Autodesk Fusion 360 part; units mm, degrees
(part 4 of 6)
sketch "Sketch2" plane through (0, 0, 0) normal (0, 0, -1) x (1, 0, 0)
  line L0 (-67.0711, -60) -> (-70, -62.9289)
  line L1 (-70, -62.9289) -> (-70, -57.0711)
  line L2 (-70, -57.0711) -> (-67.0711, -60)
  line L3 (-62.9289, -60) -> (-60, -57.0711)
  line L4 (-60, -57.0711) -> (-57.0711, -60)
  line L5 (-57.0711, -60) -> (-60, -62.9289)
  line L6 (-60, -62.9289) -> (-62.9289, -60)
  line L7 (-60, -67.0711) -> (-57.0711, -70)
  line L8 (-57.0711, -70) -> (-62.9289, -70)
  line L9 (-62.9289, -70) -> (-60, -67.0711)
  line L10 (-52.9289, -70) -> (-50, -67.0711)
  line L11 (-50, -67.0711) -> (-47.0711, -70)
  line L12 (-47.0711, -70) -> (-52.9289, -70)
  line L13 (-42.9289, -70) -> (-40, -67.0711)
  line L14 (-40, -67.0711) -> (-37.0711, -70)
  line L15 (-37.0711, -70) -> (-42.9289, -70)
  line L16 (-32.9289, -70) -> (-30, -67.0711)
  line L17 (-30, -67.0711) -> (-27.0711, -70)
  line L18 (-27.0711, -70) -> (-32.9289, -70)
  line L19 (-22.9289, -70) -> (-20, -67.0711)
  line L20 (-20, -67.0711) -> (-17.0711, -70)
  line L21 (-17.0711, -70) -> (-22.9289, -70)
  line L22 (-12.9289, -70) -> (-10, -67.0711)
  line L23 (-10, -67.0711) -> (-7.0711, -70)
  line L24 (-7.0711, -70) -> (-12.9289, -70)
  line L25 (-2.9289, -70) -> (0, -67.0711)
  line L26 (0, -67.0711) -> (2.9289, -70)
  line L27 (2.9289, -70) -> (-2.9289, -70)
  line L28 (7.0711, -70) -> (10, -67.0711)
  line L29 (10, -67.0711) -> (12.9289, -70)
  line L30 (12.9289, -70) -> (7.0711, -70)
  line L31 (17.0711, -70) -> (20, -67.0711)
  line L32 (20, -67.0711) -> (22.9289, -70)
  line L33 (22.9289, -70) -> (17.0711, -70)
  line L34 (27.0711, -70) -> (30, -67.0711)
  line L35 (30, -67.0711) -> (32.9289, -70)
  line L36 (32.9289, -70) -> (27.0711, -70)
  line L37 (37.0711, -70) -> (40, -67.0711)
  line L38 (40, -67.0711) -> (42.9289, -70)
  line L39 (42.9289, -70) -> (37.0711, -70)
  line L40 (47.0711, -70) -> (50, -67.0711)
  line L41 (50, -67.0711) -> (52.9289, -70)
  line L42 (52.9289, -70) -> (47.0711, -70)
  line L43 (57.0711, -70) -> (60, -67.0711)
  line L44 (60, -67.0711) -> (62.9289, -70)
  line L45 (62.9289, -70) -> (57.0711, -70)
  line L46 (67.0711, -70) -> (70, -67.0711)
  line L47 (70, -67.0711) -> (70, -70)
  line L48 (70, -70) -> (67.0711, -70)
  line L49 (70, -62.9289) -> (67.0711, -60)
  line L50 (67.0711, -60) -> (70, -57.0711)
  line L51 (70, -57.0711) -> (70, -62.9289)
  line L52 (70, -52.9289) -> (67.0711, -50)
  line L53 (67.0711, -50) -> (70, -47.0711)
  line L54 (70, -47.0711) -> (70, -52.9289)
  line L55 (70, -42.9289) -> (67.0711, -40)
  line L56 (67.0711, -40) -> (70, -37.0711)
  line L57 (70, -37.0711) -> (70, -42.9289)
  line L58 (70, -32.9289) -> (67.0711, -30)
  line L59 (67.0711, -30) -> (70, -27.0711)
  line L60 (70, -27.0711) -> (70, -32.9289)
  line L61 (70, -22.9289) -> (67.0711, -20)
  line L62 (67.0711, -20) -> (70, -17.0711)
  line L63 (70, -17.0711) -> (70, -22.9289)
  line L64 (70, -12.9289) -> (67.0711, -10)
  line L65 (67.0711, -10) -> (70, -7.0711)
  line L66 (70, -7.0711) -> (70, -12.9289)
  line L67 (70, -2.9289) -> (67.0711, 0)
  line L68 (67.0711, 0) -> (70, 2.9289)
  line L69 (70, 2.9289) -> (70, -2.9289)
  line L70 (70, 7.0711) -> (67.0711, 10)
  line L71 (67.0711, 10) -> (70, 12.9289)
  line L72 (70, 12.9289) -> (70, 7.0711)
  line L73 (70, 17.0711) -> (67.0711, 20)
  line L74 (67.0711, 20) -> (70, 22.9289)
  line L75 (70, 22.9289) -> (70, 17.0711)
  line L76 (70, 27.0711) -> (67.0711, 30)
  line L77 (67.0711, 30) -> (70, 32.9289)
  line L78 (70, 32.9289) -> (70, 27.0711)
  line L79 (70, 37.0711) -> (67.0711, 40)
  line L80 (67.0711, 40) -> (70, 42.9289)
  line L81 (70, 42.9289) -> (70, 37.0711)
  line L82 (70, 47.0711) -> (67.0711, 50)
  line L83 (67.0711, 50) -> (70, 52.9289)
  line L84 (70, 52.9289) -> (70, 47.0711)
  line L85 (70, 57.0711) -> (67.0711, 60)
  line L86 (67.0711, 60) -> (70, 62.9289)
  line L87 (70, 62.9289) -> (70, 57.0711)
  line L88 (70, 67.0711) -> (67.0711, 70)
  line L89 (67.0711, 70) -> (70, 70)
  line L90 (70, 70) -> (70, 67.0711)
  line L91 (62.9289, 70) -> (60, 67.0711)
  line L92 (60, 67.0711) -> (57.0711, 70)
  line L93 (57.0711, 70) -> (62.9289, 70)
  line L94 (52.9289, 70) -> (50, 67.0711)
  line L95 (50, 67.0711) -> (47.0711, 70)
  line L96 (47.0711, 70) -> (52.9289, 70)
  line L97 (42.9289, 70) -> (40, 67.0711)
  line L98 (40, 67.0711) -> (37.0711, 70)
  line L99 (37.0711, 70) -> (42.9289, 70)
  line L100 (32.9289, 70) -> (30, 67.0711)
  line L101 (30, 67.0711) -> (27.0711, 70)
  line L102 (27.0711, 70) -> (32.9289, 70)
  line L103 (22.9289, 70) -> (20, 67.0711)
  line L104 (20, 67.0711) -> (17.0711, 70)
  line L105 (17.0711, 70) -> (22.9289, 70)
  line L106 (12.9289, 70) -> (10, 67.0711)
  line L107 (10, 67.0711) -> (7.0711, 70)
  line L108 (7.0711, 70) -> (12.9289, 70)
  line L109 (2.9289, 70) -> (0, 67.0711)
  line L110 (0, 67.0711) -> (-2.9289, 70)
  line L111 (-2.9289, 70) -> (2.9289, 70)
  line L112 (-7.0711, 70) -> (-10, 67.0711)
  line L113 (-10, 67.0711) -> (-12.9289, 70)
  line L114 (-12.9289, 70) -> (-7.0711, 70)
  line L115 (-17.0711, 70) -> (-20, 67.0711)
  line L116 (-20, 67.0711) -> (-22.9289, 70)
  line L117 (-22.9289, 70) -> (-17.0711, 70)
  line L118 (-27.0711, 70) -> (-30, 67.0711)
  line L119 (-30, 67.0711) -> (-32.9289, 70)
  line L120 (-32.9289, 70) -> (-27.0711, 70)
  line L121 (-37.0711, 70) -> (-40, 67.0711)
  line L122 (-40, 67.0711) -> (-42.9289, 70)
  line L123 (-42.9289, 70) -> (-37.0711, 70)
  line L124 (-47.0711, 70) -> (-50, 67.0711)
  line L125 (-50, 67.0711) -> (-52.9289, 70)
  line L126 (-52.9289, 70) -> (-47.0711, 70)
  line L127 (-57.0711, 70) -> (-60, 67.0711)
  line L128 (-60, 67.0711) -> (-62.9289, 70)
  line L129 (-62.9289, 70) -> (-57.0711, 70)
  line L130 (-67.0711, 70) -> (-70, 67.0711)
  line L131 (-70, 67.0711) -> (-70, 70)
  line L132 (-70, 70) -> (-67.0711, 70)
  line L133 (-70, 62.9289) -> (-67.0711, 60)
  line L134 (-67.0711, 60) -> (-70, 57.0711)
  line L135 (-70, 57.0711) -> (-70, 62.9289)
  line L136 (-70, 52.9289) -> (-67.0711, 50)
  line L137 (-67.0711, 50) -> (-70, 47.0711)
  line L138 (-70, 47.0711) -> (-70, 52.9289)
  line L139 (-70, 42.9289) -> (-67.0711, 40)
  line L140 (-67.0711, 40) -> (-70, 37.0711)
  line L141 (-70, 37.0711) -> (-70, 42.9289)
  line L142 (-70, 32.9289) -> (-67.0711, 30)
  line L143 (-67.0711, 30) -> (-70, 27.0711)
  line L144 (-70, 27.0711) -> (-70, 32.9289)
  line L145 (-70, 22.9289) -> (-67.0711, 20)
  line L146 (-67.0711, 20) -> (-70, 17.0711)
  line L147 (-70, 17.0711) -> (-70, 22.9289)
  line L148 (-70, 12.9289) -> (-67.0711, 10)
  line L149 (-67.0711, 10) -> (-70, 7.0711)
  line L150 (-70, 7.0711) -> (-70, 12.9289)
  line L151 (-70, 2.9289) -> (-67.0711, 0)
  line L152 (-67.0711, 0) -> (-70, -2.9289)
  line L153 (-70, -2.9289) -> (-70, 2.9289)
  line L154 (-70, -7.0711) -> (-67.0711, -10)
  line L155 (-67.0711, -10) -> (-70, -12.9289)
  line L156 (-70, -12.9289) -> (-70, -7.0711)
  line L157 (-70, -17.0711) -> (-67.0711, -20)
  line L158 (-67.0711, -20) -> (-70, -22.9289)
  line L159 (-70, -22.9289) -> (-70, -17.0711)
  line L160 (-70, -27.0711) -> (-67.0711, -30)
  line L161 (-67.0711, -30) -> (-70, -32.9289)
  line L162 (-70, -32.9289) -> (-70, -27.0711)
  line L163 (-70, -37.0711) -> (-67.0711, -40)
  line L164 (-67.0711, -40) -> (-70, -42.9289)
  line L165 (-70, -42.9289) -> (-70, -37.0711)
  line L166 (-17.0711, 40) -> (-20, 37.0711)
  line L167 (-20, 37.0711) -> (-22.9289, 40)
  line L168 (-22.9289, 40) -> (-20, 42.9289)
  line L169 (-20, 42.9289) -> (-17.0711, 40)
  line L170 (-27.0711, 40) -> (-30, 37.0711)
  line L171 (-30, 37.0711) -> (-32.9289, 40)
  line L172 (-32.9289, 40) -> (-30, 42.9289)
  line L173 (-30, 42.9289) -> (-27.0711, 40)
  line L174 (-37.0711, 40) -> (-40, 37.0711)
  line L175 (-40, 37.0711) -> (-42.9289, 40)
  line L176 (-42.9289, 40) -> (-40, 42.9289)
  line L177 (-40, 42.9289) -> (-37.0711, 40)
  line L178 (-37.0711, 30) -> (-40, 27.0711)
  line L179 (-40, 27.0711) -> (-42.9289, 30)
  line L180 (-42.9289, 30) -> (-40, 32.9289)
  line L181 (-40, 32.9289) -> (-37.0711, 30)
  line L182 (-37.0711, 20) -> (-40, 17.0711)
  line L183 (-40, 17.0711) -> (-42.9289, 20)
  line L184 (-42.9289, 20) -> (-40, 22.9289)
  line L185 (-40, 22.9289) -> (-37.0711, 20)
  line L186 (-37.0711, 10) -> (-40, 7.0711)
  line L187 (-40, 7.0711) -> (-42.9289, 10)
  line L188 (-42.9289, 10) -> (-40, 12.9289)
  line L189 (-40, 12.9289) -> (-37.0711, 10)
  line L190 (-37.0711, 0) -> (-40, -2.9289)
  line L191 (-40, -2.9289) -> (-42.9289, 0)
  line L192 (-42.9289, 0) -> (-40, 2.9289)
  line L193 (-40, 2.9289) -> (-37.0711, 0)
  line L194 (-37.0711, -10) -> (-40, -12.9289)
  line L195 (-40, -12.9289) -> (-42.9289, -10)
  line L196 (-42.9289, -10) -> (-40, -7.0711)
  line L197 (-40, -7.0711) -> (-37.0711, -10)
  line L198 (-37.0711, -20) -> (-40, -22.9289)
  line L199 (-40, -22.9289) -> (-42.9289, -20)
  line L200 (-42.9289, -20) -> (-40, -17.0711)
  line L201 (-40, -17.0711) -> (-37.0711, -20)
  line L202 (-37.0711, -30) -> (-40, -32.9289)
  line L203 (-40, -32.9289) -> (-42.9289, -30)
  line L204 (-42.9289, -30) -> (-40, -27.0711)
  line L205 (-40, -27.0711) -> (-37.0711, -30)
  line L206 (-27.0711, -20) -> (-30, -22.9289)
  line L207 (-30, -22.9289) -> (-32.9289, -20)
  line L208 (-32.9289, -20) -> (-30, -17.0711)
  line L209 (-30, -17.0711) -> (-27.0711, -20)
  line L210 (-17.0711, -20) -> (-20, -22.9289)
  line L211 (-20, -22.9289) -> (-22.9289, -20)
  line L212 (-22.9289, -20) -> (-20, -17.0711)
  line L213 (-20, -17.0711) -> (-17.0711, -20)
  line L214 (-7.0711, -30) -> (-10, -32.9289)
  line L215 (-10, -32.9289) -> (-12.9289, -30)
  line L216 (-12.9289, -30) -> (-10, -27.0711)
  line L217 (-10, -27.0711) -> (-7.0711, -30)
  line L218 (2.9289, -30) -> (0, -32.9289)
  line L219 (0, -32.9289) -> (-2.9289, -30)
  line L220 (-2.9289, -30) -> (0, -27.0711)
  line L221 (0, -27.0711) -> (2.9289, -30)
  line L222 (12.9289, -30) -> (10, -32.9289)
  line L223 (10, -32.9289) -> (7.0711, -30)
  line L224 (7.0711, -30) -> (10, -27.0711)
  line L225 (10, -27.0711) -> (12.9289, -30)
  line L226 (22.9289, -30) -> (20, -32.9289)
  line L227 (20, -32.9289) -> (17.0711, -30)
  line L228 (17.0711, -30) -> (20, -27.0711)
  line L229 (20, -27.0711) -> (22.9289, -30)
  line L230 (32.9289, -30) -> (30, -32.9289)
  line L231 (30, -32.9289) -> (27.0711, -30)
  line L232 (27.0711, -30) -> (30, -27.0711)
  line L233 (30, -27.0711) -> (32.9289, -30)
  line L234 (32.9289, -10) -> (30, -12.9289)
  line L235 (30, -12.9289) -> (27.0711, -10)
  line L236 (27.0711, -10) -> (30, -7.0711)
  line L237 (30, -7.0711) -> (32.9289, -10)
  line L238 (32.9289, -20) -> (30, -22.9289)
  line L239 (30, -22.9289) -> (27.0711, -20)
  line L240 (27.0711, -20) -> (30, -17.0711)
  line L241 (30, -17.0711) -> (32.9289, -20)
  line L242 (32.9289, 10) -> (30, 7.0711)
  line L243 (30, 7.0711) -> (27.0711, 10)
  line L244 (27.0711, 10) -> (30, 12.9289)
  line L245 (30, 12.9289) -> (32.9289, 10)
  line L246 (32.9289, 20) -> (30, 17.0711)
  line L247 (30, 17.0711) -> (27.0711, 20)
  line L248 (27.0711, 20) -> (30, 22.9289)
  line L249 (30, 22.9289) -> (32.9289, 20)
  line L250 (32.9289, 0) -> (30, -2.9289)
  line L251 (30, -2.9289) -> (27.0711, 0)
  line L252 (27.0711, 0) -> (30, 2.9289)
  line L253 (30, 2.9289) -> (32.9289, 0)
  line L254 (32.9289, 30) -> (30, 27.0711)
  line L255 (30, 27.0711) -> (27.0711, 30)
  line L256 (27.0711, 30) -> (30, 32.9289)
  line L257 (30, 32.9289) -> (32.9289, 30)
  line L258 (12.9289, 30) -> (10, 27.0711)
  line L259 (10, 27.0711) -> (7.0711, 30)
  line L260 (7.0711, 30) -> (10, 32.9289)
  line L261 (10, 32.9289) -> (12.9289, 30)
  line L262 (2.9289, 30) -> (0, 27.0711)
  line L263 (0, 27.0711) -> (-2.9289, 30)
  line L264 (-2.9289, 30) -> (0, 32.9289)
  line L265 (0, 32.9289) -> (2.9289, 30)
  line L266 (-17.0711, 30) -> (-20, 27.0711)
  line L267 (-20, 27.0711) -> (-22.9289, 30)
  line L268 (-22.9289, 30) -> (-20, 32.9289)
  line L269 (-20, 32.9289) -> (-17.0711, 30)
  line L270 (-7.0711, 30) -> (-10, 27.0711)
  line L271 (-10, 27.0711) -> (-12.9289, 30)
  line L272 (-12.9289, 30) -> (-10, 32.9289)
  line L273 (-10, 32.9289) -> (-7.0711, 30)
  line L274 (-27.0711, 20) -> (-30, 17.0711)
  line L275 (-30, 17.0711) -> (-32.9289, 20)
  line L276 (-32.9289, 20) -> (-30, 22.9289)
  line L277 (-30, 22.9289) -> (-27.0711, 20)
  line L278 (-27.0711, 10) -> (-30, 7.0711)
  line L279 (-30, 7.0711) -> (-32.9289, 10)
  line L280 (-32.9289, 10) -> (-30, 12.9289)
  line L281 (-30, 12.9289) -> (-27.0711, 10)
  line L282 (-27.0711, 30) -> (-30, 27.0711)
  line L283 (-30, 27.0711) -> (-32.9289, 30)
  line L284 (-32.9289, 30) -> (-30, 32.9289)
  line L285 (-30, 32.9289) -> (-27.0711, 30)
  line L286 (-27.0711, 0) -> (-30, -2.9289)
  line L287 (-30, -2.9289) -> (-32.9289, 0)
  line L288 (-32.9289, 0) -> (-30, 2.9289)
  line L289 (-30, 2.9289) -> (-27.0711, 0)
  line L290 (-27.0711, -10) -> (-30, -12.9289)
  line L291 (-30, -12.9289) -> (-32.9289, -10)
  line L292 (-32.9289, -10) -> (-30, -7.0711)
  line L293 (-30, -7.0711) -> (-27.0711, -10)
  line L294 (-17.0711, -10) -> (-20, -12.9289)
  line L295 (-20, -12.9289) -> (-22.9289, -10)
  line L296 (-22.9289, -10) -> (-20, -7.0711)
  line L297 (-20, -7.0711) -> (-17.0711, -10)
  line L298 (-7.0711, -20) -> (-10, -22.9289)
  line L299 (-10, -22.9289) -> (-12.9289, -20)
  line L300 (-12.9289, -20) -> (-10, -17.0711)
  line L301 (-10, -17.0711) -> (-7.0711, -20)
  line L302 (2.9289, -20) -> (0, -22.9289)
  line L303 (0, -22.9289) -> (-2.9289, -20)
  line L304 (-2.9289, -20) -> (0, -17.0711)
  line L305 (0, -17.0711) -> (2.9289, -20)
  line L306 (12.9289, -20) -> (10, -22.9289)
  line L307 (10, -22.9289) -> (7.0711, -20)
  line L308 (7.0711, -20) -> (10, -17.0711)
  line L309 (10, -17.0711) -> (12.9289, -20)
  line L310 (22.9289, -20) -> (20, -22.9289)
  line L311 (20, -22.9289) -> (17.0711, -20)
  line L312 (17.0711, -20) -> (20, -17.0711)
  line L313 (20, -17.0711) -> (22.9289, -20)
  line L314 (22.9289, -10) -> (20, -12.9289)
  line L315 (20, -12.9289) -> (17.0711, -10)
  line L316 (17.0711, -10) -> (20, -7.0711)
  line L317 (20, -7.0711) -> (22.9289, -10)
  line L318 (22.9289, 10) -> (20, 7.0711)
  line L319 (20, 7.0711) -> (17.0711, 10)
  line L320 (17.0711, 10) -> (20, 12.9289)
  line L321 (20, 12.9289) -> (22.9289, 10)
  line L322 (22.9289, 20) -> (20, 17.0711)
  line L323 (20, 17.0711) -> (17.0711, 20)
  line L324 (17.0711, 20) -> (20, 22.9289)
  line L325 (20, 22.9289) -> (22.9289, 20)
  line L326 (22.9289, 0) -> (20, -2.9289)
  line L327 (20, -2.9289) -> (17.0711, 0)
  line L328 (17.0711, 0) -> (20, 2.9289)
  line L329 (20, 2.9289) -> (22.9289, 0)
  line L330 (22.9289, 30) -> (20, 27.0711)
  line L331 (20, 27.0711) -> (17.0711, 30)
  line L332 (17.0711, 30) -> (20, 32.9289)
  line L333 (20, 32.9289) -> (22.9289, 30)
  line L334 (12.9289, 20) -> (10, 17.0711)
  line L335 (10, 17.0711) -> (7.0711, 20)
  line L336 (7.0711, 20) -> (10, 22.9289)
  line L337 (10, 22.9289) -> (12.9289, 20)
  line L338 (2.9289, 20) -> (0, 17.0711)
  line L339 (0, 17.0711) -> (-2.9289, 20)
  line L340 (-2.9289, 20) -> (0, 22.9289)
  line L341 (0, 22.9289) -> (2.9289, 20)
  line L342 (-7.0711, 20) -> (-10, 17.0711)
  line L343 (-10, 17.0711) -> (-12.9289, 20)
  line L344 (-12.9289, 20) -> (-10, 22.9289)
  line L345 (-10, 22.9289) -> (-7.0711, 20)
  line L346 (-17.0711, 20) -> (-20, 17.0711)
  line L347 (-20, 17.0711) -> (-22.9289, 20)
  line L348 (-22.9289, 20) -> (-20, 22.9289)
  line L349 (-20, 22.9289) -> (-17.0711, 20)
  line L350 (-17.0711, 10) -> (-20, 7.0711)
  line L351 (-20, 7.0711) -> (-22.9289, 10)
  line L352 (-22.9289, 10) -> (-20, 12.9289)
  line L353 (-20, 12.9289) -> (-17.0711, 10)
  line L354 (-7.0711, -10) -> (-10, -12.9289)
  line L355 (-10, -12.9289) -> (-12.9289, -10)
  line L356 (-12.9289, -10) -> (-10, -7.0711)
  line L357 (-10, -7.0711) -> (-7.0711, -10)
  line L358 (-49, -66.6569) -> (-49, -63.3431)
  line L359 (-49, -63.3431) -> (-46.6569, -61)
  line L360 (-46.6569, -61) -> (-43.3431, -61)
  line L361 (-43.3431, -61) -> (-41, -63.3431)
  line L362 (-41, -63.3431) -> (-41, -66.6569)
  line L363 (-41, -66.6569) -> (-43.3431, -69)
  line L364 (-43.3431, -69) -> (-46.6569, -69)
  line L365 (-46.6569, -69) -> (-49, -66.6569)
  line L366 (-19, -66.6569) -> (-19, -63.3431)
  line L367 (-19, -63.3431) -> (-16.6569, -61)
  line L368 (-16.6569, -61) -> (-13.3431, -61)
  line L369 (-13.3431, -61) -> (-11, -63.3431)
  line L370 (-11, -63.3431) -> (-11, -66.6569)
  line L371 (-11, -66.6569) -> (-13.3431, -69)
  line L372 (-13.3431, -69) -> (-16.6569, -69)
  line L373 (-16.6569, -69) -> (-19, -66.6569)
  line L374 (-59, -66.6569) -> (-59, -63.3431)
  line L375 (-59, -63.3431) -> (-56.6569, -61)
  line L376 (-56.6569, -61) -> (-53.3431, -61)
  line L377 (-53.3431, -61) -> (-51, -63.3431)
  line L378 (-51, -63.3431) -> (-51, -66.6569)
  line L379 (-51, -66.6569) -> (-53.3431, -69)
  line L380 (-53.3431, -69) -> (-56.6569, -69)
  line L381 (-56.6569, -69) -> (-59, -66.6569)
  line L382 (-17.0711, 0) -> (-20, -2.9289)
  line L383 (-20, -2.9289) -> (-22.9289, 0)
  line L384 (-22.9289, 0) -> (-20, 2.9289)
  line L385 (-20, 2.9289) -> (-17.0711, 0)
  line L386 (-59, -26.6569) -> (-59, -23.3431)
  line L387 (-59, -23.3431) -> (-56.6569, -21)
  line L388 (-56.6569, -21) -> (-53.3431, -21)
  line L389 (-53.3431, -21) -> (-51, -23.3431)
  line L390 (-51, -23.3431) -> (-51, -26.6569)
  line L391 (-51, -26.6569) -> (-53.3431, -29)
  line L392 (-53.3431, -29) -> (-56.6569, -29)
  line L393 (-56.6569, -29) -> (-59, -26.6569)
  line L394 (-29, -66.6569) -> (-29, -63.3431)
  line L395 (-29, -63.3431) -> (-26.6569, -61)
  line L396 (-26.6569, -61) -> (-23.3431, -61)
  line L397 (-23.3431, -61) -> (-21, -63.3431)
  line L398 (-21, -63.3431) -> (-21, -66.6569)
  line L399 (-21, -66.6569) -> (-23.3431, -69)
  line L400 (-23.3431, -69) -> (-26.6569, -69)
  line L401 (-26.6569, -69) -> (-29, -66.6569)
  line L402 (41, -66.6569) -> (41, -63.3431)
  line L403 (41, -63.3431) -> (43.3431, -61)
  line L404 (43.3431, -61) -> (46.6569, -61)
  line L405 (46.6569, -61) -> (49, -63.3431)
  line L406 (49, -63.3431) -> (49, -66.6569)
  line L407 (49, -66.6569) -> (46.6569, -69)
  line L408 (46.6569, -69) -> (43.3431, -69)
  line L409 (43.3431, -69) -> (41, -66.6569)
  line L410 (11, -56.6569) -> (11, -53.3431)
  line L411 (11, -53.3431) -> (13.3431, -51)
  line L412 (13.3431, -51) -> (16.6569, -51)
  line L413 (16.6569, -51) -> (19, -53.3431)
  line L414 (19, -53.3431) -> (19, -56.6569)
  line L415 (19, -56.6569) -> (16.6569, -59)
  line L416 (16.6569, -59) -> (13.3431, -59)
  line L417 (13.3431, -59) -> (11, -56.6569)
  line L418 (21, -56.6569) -> (21, -53.3431)
  line L419 (21, -53.3431) -> (23.3431, -51)
  line L420 (23.3431, -51) -> (26.6569, -51)
  line L421 (26.6569, -51) -> (29, -53.3431)
  line L422 (29, -53.3431) -> (29, -56.6569)
  line L423 (29, -56.6569) -> (26.6569, -59)
  line L424 (26.6569, -59) -> (23.3431, -59)
  line L425 (23.3431, -59) -> (21, -56.6569)
  line L426 (-29, -46.6569) -> (-29, -43.3431)
  line L427 (-29, -43.3431) -> (-26.6569, -41)
  line L428 (-26.6569, -41) -> (-23.3431, -41)
  line L429 (-23.3431, -41) -> (-21, -43.3431)
  line L430 (-21, -43.3431) -> (-21, -46.6569)
  line L431 (-21, -46.6569) -> (-23.3431, -49)
  line L432 (-23.3431, -49) -> (-26.6569, -49)
  line L433 (-26.6569, -49) -> (-29, -46.6569)
  line L434 (-29, -26.6569) -> (-29, -23.3431)
  line L435 (-29, -23.3431) -> (-26.6569, -21)
  line L436 (-26.6569, -21) -> (-23.3431, -21)
  line L437 (-23.3431, -21) -> (-21, -23.3431)
  line L438 (-21, -23.3431) -> (-21, -26.6569)
  line L439 (-21, -26.6569) -> (-23.3431, -29)
  line L440 (-23.3431, -29) -> (-26.6569, -29)
  line L441 (-26.6569, -29) -> (-29, -26.6569)
  line L442 (-19, -26.6569) -> (-19, -23.3431)
  line L443 (-19, -23.3431) -> (-16.6569, -21)
  line L444 (-16.6569, -21) -> (-13.3431, -21)
  line L445 (-13.3431, -21) -> (-11, -23.3431)
  line L446 (-11, -23.3431) -> (-11, -26.6569)
  line L447 (-11, -26.6569) -> (-13.3431, -29)
  line L448 (-13.3431, -29) -> (-16.6569, -29)
  line L449 (-16.6569, -29) -> (-19, -26.6569)
  line L450 (-39, -26.6569) -> (-39, -23.3431)
  line L451 (-39, -23.3431) -> (-36.6569, -21)
  line L452 (-36.6569, -21) -> (-33.3431, -21)
  line L453 (-33.3431, -21) -> (-31, -23.3431)
  line L454 (-31, -23.3431) -> (-31, -26.6569)
  line L455 (-31, -26.6569) -> (-33.3431, -29)
  line L456 (-33.3431, -29) -> (-36.6569, -29)
  line L457 (-36.6569, -29) -> (-39, -26.6569)
  line L458 (-19, -46.6569) -> (-19, -43.3431)
  line L459 (-19, -43.3431) -> (-16.6569, -41)
  line L460 (-16.6569, -41) -> (-13.3431, -41)
  line L461 (-13.3431, -41) -> (-11, -43.3431)
  line L462 (-11, -43.3431) -> (-11, -46.6569)
  line L463 (-11, -46.6569) -> (-13.3431, -49)
  line L464 (-13.3431, -49) -> (-16.6569, -49)
  line L465 (-16.6569, -49) -> (-19, -46.6569)
  line L466 (-49, -26.6569) -> (-49, -23.3431)
  line L467 (-49, -23.3431) -> (-46.6569, -21)
  line L468 (-46.6569, -21) -> (-43.3431, -21)
  line L469 (-43.3431, -21) -> (-41, -23.3431)
  line L470 (-41, -23.3431) -> (-41, -26.6569)
  line L471 (-41, -26.6569) -> (-43.3431, -29)
  line L472 (-43.3431, -29) -> (-46.6569, -29)
  line L473 (-46.6569, -29) -> (-49, -26.6569)
  line L474 (-49, -46.6569) -> (-49, -43.3431)
  line L475 (-49, -43.3431) -> (-46.6569, -41)
  line L476 (-46.6569, -41) -> (-43.3431, -41)
  line L477 (-43.3431, -41) -> (-41, -43.3431)
  line L478 (-41, -43.3431) -> (-41, -46.6569)
  line L479 (-41, -46.6569) -> (-43.3431, -49)
  line L480 (-43.3431, -49) -> (-46.6569, -49)
  line L481 (-46.6569, -49) -> (-49, -46.6569)
  line L482 (-39, -46.6569) -> (-39, -43.3431)
  line L483 (-39, -43.3431) -> (-36.6569, -41)
  line L484 (-36.6569, -41) -> (-33.3431, -41)
  line L485 (-33.3431, -41) -> (-31, -43.3431)
  line L486 (-31, -43.3431) -> (-31, -46.6569)
  line L487 (-31, -46.6569) -> (-33.3431, -49)
  line L488 (-33.3431, -49) -> (-36.6569, -49)
  line L489 (-36.6569, -49) -> (-39, -46.6569)
  line L490 (-59, -46.6569) -> (-59, -43.3431)
  line L491 (-59, -43.3431) -> (-56.6569, -41)
  line L492 (-56.6569, -41) -> (-53.3431, -41)
  line L493 (-53.3431, -41) -> (-51, -43.3431)
  line L494 (-51, -43.3431) -> (-51, -46.6569)
  line L495 (-51, -46.6569) -> (-53.3431, -49)
  line L496 (-53.3431, -49) -> (-56.6569, -49)
  line L497 (-56.6569, -49) -> (-59, -46.6569)
  line L498 (61, -56.6569) -> (61, -53.3431)
  line L499 (61, -53.3431) -> (63.3431, -51)
  line L500 (63.3431, -51) -> (66.6569, -51)
  line L501 (66.6569, -51) -> (69, -53.3431)
  line L502 (69, -53.3431) -> (69, -56.6569)
  line L503 (69, -56.6569) -> (66.6569, -59)
  line L504 (66.6569, -59) -> (63.3431, -59)
  line L505 (63.3431, -59) -> (61, -56.6569)
  line L506 (-69, -46.6569) -> (-69, -43.3431)
  line L507 (-69, -43.3431) -> (-66.6569, -41)
  line L508 (-66.6569, -41) -> (-63.3431, -41)
  line L509 (-63.3431, -41) -> (-61, -43.3431)
  line L510 (-61, -43.3431) -> (-61, -46.6569)
  line L511 (-61, -46.6569) -> (-63.3431, -49)
  line L512 (-63.3431, -49) -> (-66.6569, -49)
  line L513 (-66.6569, -49) -> (-69, -46.6569)
  line L514 (51, -56.6569) -> (51, -53.3431)
  line L515 (51, -53.3431) -> (53.3431, -51)
  line L516 (53.3431, -51) -> (56.6569, -51)
  line L517 (56.6569, -51) -> (59, -53.3431)
  line L518 (59, -53.3431) -> (59, -56.6569)
  line L519 (59, -56.6569) -> (56.6569, -59)
  line L520 (56.6569, -59) -> (53.3431, -59)
  line L521 (53.3431, -59) -> (51, -56.6569)
  line L522 (41, -56.6569) -> (41, -53.3431)
  line L523 (41, -53.3431) -> (43.3431, -51)
  line L524 (43.3431, -51) -> (46.6569, -51)
  line L525 (46.6569, -51) -> (49, -53.3431)
  line L526 (49, -53.3431) -> (49, -56.6569)
  line L527 (49, -56.6569) -> (46.6569, -59)
  line L528 (46.6569, -59) -> (43.3431, -59)
  line L529 (43.3431, -59) -> (41, -56.6569)
  line L530 (31, -56.6569) -> (31, -53.3431)
  line L531 (31, -53.3431) -> (33.3431, -51)
  line L532 (33.3431, -51) -> (36.6569, -51)
  line L533 (36.6569, -51) -> (39, -53.3431)
  line L534 (39, -53.3431) -> (39, -56.6569)
  line L535 (39, -56.6569) -> (36.6569, -59)
  line L536 (36.6569, -59) -> (33.3431, -59)
  line L537 (33.3431, -59) -> (31, -56.6569)
  line L538 (1, -56.6569) -> (1, -53.3431)
  line L539 (1, -53.3431) -> (3.3431, -51)
  line L540 (3.3431, -51) -> (6.6569, -51)
  line L541 (6.6569, -51) -> (9, -53.3431)
  line L542 (9, -53.3431) -> (9, -56.6569)
  line L543 (9, -56.6569) -> (6.6569, -59)
  line L544 (6.6569, -59) -> (3.3431, -59)
  line L545 (3.3431, -59) -> (1, -56.6569)
  line L546 (51, -66.6569) -> (51, -63.3431)
  line L547 (51, -63.3431) -> (53.3431, -61)
  line L548 (53.3431, -61) -> (56.6569, -61)
  line L549 (56.6569, -61) -> (59, -63.3431)
  line L550 (59, -63.3431) -> (59, -66.6569)
  line L551 (59, -66.6569) -> (56.6569, -69)
  line L552 (56.6569, -69) -> (53.3431, -69)
  line L553 (53.3431, -69) -> (51, -66.6569)
  line L554 (61, -66.6569) -> (61, -63.3431)
  line L555 (61, -63.3431) -> (63.3431, -61)
  line L556 (63.3431, -61) -> (66.6569, -61)
  line L557 (66.6569, -61) -> (69, -63.3431)
  line L558 (69, -63.3431) -> (69, -66.6569)
  line L559 (69, -66.6569) -> (66.6569, -69)
  line L560 (66.6569, -69) -> (63.3431, -69)
  line L561 (63.3431, -69) -> (61, -66.6569)
  line L562 (-59, -56.6569) -> (-59, -53.3431)
  line L563 (-59, -53.3431) -> (-56.6569, -51)
  line L564 (-56.6569, -51) -> (-53.3431, -51)
  line L565 (-53.3431, -51) -> (-51, -53.3431)
  line L566 (-51, -53.3431) -> (-51, -56.6569)
  line L567 (-51, -56.6569) -> (-53.3431, -59)
  line L568 (-53.3431, -59) -> (-56.6569, -59)
  line L569 (-56.6569, -59) -> (-59, -56.6569)
  line L570 (-69, -56.6569) -> (-69, -53.3431)
  line L571 (-69, -53.3431) -> (-66.6569, -51)
  line L572 (-66.6569, -51) -> (-63.3431, -51)
  line L573 (-63.3431, -51) -> (-61, -53.3431)
  line L574 (-61, -53.3431) -> (-61, -56.6569)
  line L575 (-61, -56.6569) -> (-63.3431, -59)
  line L576 (-63.3431, -59) -> (-66.6569, -59)
  line L577 (-66.6569, -59) -> (-69, -56.6569)
  line L578 (-49, -56.6569) -> (-49, -53.3431)
  line L579 (-49, -53.3431) -> (-46.6569, -51)
  line L580 (-46.6569, -51) -> (-43.3431, -51)
  line L581 (-43.3431, -51) -> (-41, -53.3431)
  line L582 (-41, -53.3431) -> (-41, -56.6569)
  line L583 (-41, -56.6569) -> (-43.3431, -59)
  line L584 (-43.3431, -59) -> (-46.6569, -59)
  line L585 (-46.6569, -59) -> (-49, -56.6569)
  line L586 (-29, -56.6569) -> (-29, -53.3431)
  line L587 (-29, -53.3431) -> (-26.6569, -51)
  line L588 (-26.6569, -51) -> (-23.3431, -51)
  line L589 (-23.3431, -51) -> (-21, -53.3431)
  line L590 (-21, -53.3431) -> (-21, -56.6569)
  line L591 (-21, -56.6569) -> (-23.3431, -59)
  line L592 (-23.3431, -59) -> (-26.6569, -59)
  line L593 (-26.6569, -59) -> (-29, -56.6569)
  line L594 (-39, -56.6569) -> (-39, -53.3431)
  line L595 (-39, -53.3431) -> (-36.6569, -51)
  line L596 (-36.6569, -51) -> (-33.3431, -51)
  line L597 (-33.3431, -51) -> (-31, -53.3431)
  line L598 (-31, -53.3431) -> (-31, -56.6569)
  line L599 (-31, -56.6569) -> (-33.3431, -59)
  line L600 (-33.3431, -59) -> (-36.6569, -59)
  line L601 (-36.6569, -59) -> (-39, -56.6569)
  line L602 (-9, -56.6569) -> (-9, -53.3431)
  line L603 (-9, -53.3431) -> (-6.6569, -51)
  line L604 (-6.6569, -51) -> (-3.3431, -51)
  line L605 (-3.3431, -51) -> (-1, -53.3431)
  line L606 (-1, -53.3431) -> (-1, -56.6569)
  line L607 (-1, -56.6569) -> (-3.3431, -59)
  line L608 (-3.3431, -59) -> (-6.6569, -59)
  line L609 (-6.6569, -59) -> (-9, -56.6569)
  line L610 (-19, -56.6569) -> (-19, -53.3431)
  line L611 (-19, -53.3431) -> (-16.6569, -51)
  line L612 (-16.6569, -51) -> (-13.3431, -51)
  line L613 (-13.3431, -51) -> (-11, -53.3431)
  line L614 (-11, -53.3431) -> (-11, -56.6569)
  line L615 (-11, -56.6569) -> (-13.3431, -59)
  line L616 (-13.3431, -59) -> (-16.6569, -59)
  line L617 (-16.6569, -59) -> (-19, -56.6569)
  line L618 (21, -66.6569) -> (21, -63.3431)
  line L619 (21, -63.3431) -> (23.3431, -61)
  line L620 (23.3431, -61) -> (26.6569, -61)
  line L621 (26.6569, -61) -> (29, -63.3431)
  line L622 (29, -63.3431) -> (29, -66.6569)
  line L623 (29, -66.6569) -> (26.6569, -69)
  line L624 (26.6569, -69) -> (23.3431, -69)
  line L625 (23.3431, -69) -> (21, -66.6569)
  line L626 (31, -66.6569) -> (31, -63.3431)
  line L627 (31, -63.3431) -> (33.3431, -61)
  line L628 (33.3431, -61) -> (36.6569, -61)
  line L629 (36.6569, -61) -> (39, -63.3431)
  line L630 (39, -63.3431) -> (39, -66.6569)
  line L631 (39, -66.6569) -> (36.6569, -69)
  line L632 (36.6569, -69) -> (33.3431, -69)
  line L633 (33.3431, -69) -> (31, -66.6569)
  line L634 (11, -66.6569) -> (11, -63.3431)
  line L635 (11, -63.3431) -> (13.3431, -61)
  line L636 (13.3431, -61) -> (16.6569, -61)
  line L637 (16.6569, -61) -> (19, -63.3431)
  line L638 (19, -63.3431) -> (19, -66.6569)
  line L639 (19, -66.6569) -> (16.6569, -69)
  line L640 (16.6569, -69) -> (13.3431, -69)
  line L641 (13.3431, -69) -> (11, -66.6569)
  line L642 (1, -66.6569) -> (1, -63.3431)
  line L643 (1, -63.3431) -> (3.3431, -61)
  line L644 (3.3431, -61) -> (6.6569, -61)
  line L645 (6.6569, -61) -> (9, -63.3431)
  line L646 (9, -63.3431) -> (9, -66.6569)
  line L647 (9, -66.6569) -> (6.6569, -69)
  line L648 (6.6569, -69) -> (3.3431, -69)
  line L649 (3.3431, -69) -> (1, -66.6569)
  line L650 (-39, -66.6569) -> (-39, -63.3431)
  line L651 (-39, -63.3431) -> (-36.6569, -61)
  line L652 (-36.6569, -61) -> (-33.3431, -61)
  line L653 (-33.3431, -61) -> (-31, -63.3431)
  line L654 (-31, -63.3431) -> (-31, -66.6569)
  line L655 (-31, -66.6569) -> (-33.3431, -69)
  line L656 (-33.3431, -69) -> (-36.6569, -69)
  line L657 (-36.6569, -69) -> (-39, -66.6569)
  line L658 (-9, -66.6569) -> (-9, -63.3431)
  line L659 (-9, -63.3431) -> (-6.6569, -61)
  line L660 (-6.6569, -61) -> (-3.3431, -61)
  line L661 (-3.3431, -61) -> (-1, -63.3431)
  line L662 (-1, -63.3431) -> (-1, -66.6569)
  line L663 (-1, -66.6569) -> (-3.3431, -69)
  line L664 (-3.3431, -69) -> (-6.6569, -69)
  line L665 (-6.6569, -69) -> (-9, -66.6569)
  line L666 (62.9289, 30) -> (60, 27.0711)
  line L667 (60, 27.0711) -> (57.0711, 30)
  line L668 (57.0711, 30) -> (60, 32.9289)
  line L669 (60, 32.9289) -> (62.9289, 30)
  line L670 (-57.0711, 60) -> (-60, 57.0711)
  line L671 (-60, 57.0711) -> (-62.9289, 60)
  line L672 (-62.9289, 60) -> (-60, 62.9289)
  line L673 (-60, 62.9289) -> (-57.0711, 60)
  line L674 (-47.0711, 60) -> (-50, 57.0711)
  line L675 (-50, 57.0711) -> (-52.9289, 60)
  line L676 (-52.9289, 60) -> (-50, 62.9289)
  line L677 (-50, 62.9289) -> (-47.0711, 60)
  line L678 (-57.0711, 50) -> (-60, 47.0711)
  line L679 (-60, 47.0711) -> (-62.9289, 50)
  line L680 (-62.9289, 50) -> (-60, 52.9289)
  line L681 (-60, 52.9289) -> (-57.0711, 50)
  line L682 (-57.0711, 40) -> (-60, 37.0711)
  line L683 (-60, 37.0711) -> (-62.9289, 40)
  line L684 (-62.9289, 40) -> (-60, 42.9289)
  line L685 (-60, 42.9289) -> (-57.0711, 40)
  line L686 (-57.0711, 30) -> (-60, 27.0711)
  line L687 (-60, 27.0711) -> (-62.9289, 30)
  line L688 (-62.9289, 30) -> (-60, 32.9289)
  line L689 (-60, 32.9289) -> (-57.0711, 30)
  line L690 (-57.0711, 20) -> (-60, 17.0711)
  line L691 (-60, 17.0711) -> (-62.9289, 20)
  line L692 (-62.9289, 20) -> (-60, 22.9289)
  line L693 (-60, 22.9289) -> (-57.0711, 20)
  line L694 (-57.0711, 10) -> (-60, 7.0711)
  line L695 (-60, 7.0711) -> (-62.9289, 10)
  line L696 (-62.9289, 10) -> (-60, 12.9289)
  line L697 (-60, 12.9289) -> (-57.0711, 10)
  line L698 (-57.0711, -40) -> (-60, -42.9289)
  line L699 (-60, -42.9289) -> (-62.9289, -40)
  line L700 (-62.9289, -40) -> (-60, -37.0711)
  line L701 (-60, -37.0711) -> (-57.0711, -40)
  line L702 (-57.0711, 0) -> (-60, -2.9289)
  line L703 (-60, -2.9289) -> (-62.9289, 0)
  line L704 (-62.9289, 0) -> (-60, 2.9289)
  line L705 (-60, 2.9289) -> (-57.0711, 0)
  line L706 (-57.0711, -30) -> (-60, -32.9289)
  line L707 (-60, -32.9289) -> (-62.9289, -30)
  line L708 (-62.9289, -30) -> (-60, -27.0711)
  line L709 (-60, -27.0711) -> (-57.0711, -30)
  line L710 (-57.0711, -20) -> (-60, -22.9289)
  line L711 (-60, -22.9289) -> (-62.9289, -20)
  line L712 (-62.9289, -20) -> (-60, -17.0711)
  line L713 (-60, -17.0711) -> (-57.0711, -20)
  line L714 (-57.0711, -10) -> (-60, -12.9289)
  line L715 (-60, -12.9289) -> (-62.9289, -10)
  line L716 (-62.9289, -10) -> (-60, -7.0711)
  line L717 (-60, -7.0711) -> (-57.0711, -10)
  line L718 (12.9289, 40) -> (10, 37.0711)
  line L719 (10, 37.0711) -> (7.0711, 40)
  line L720 (7.0711, 40) -> (10, 42.9289)
  line L721 (10, 42.9289) -> (12.9289, 40)
  line L722 (32.9289, 40) -> (30, 37.0711)
  line L723 (30, 37.0711) -> (27.0711, 40)
  line L724 (27.0711, 40) -> (30, 42.9289)
  line L725 (30, 42.9289) -> (32.9289, 40)
  line L726 (22.9289, 40) -> (20, 37.0711)
  line L727 (20, 37.0711) -> (17.0711, 40)
  line L728 (17.0711, 40) -> (20, 42.9289)
  line L729 (20, 42.9289) -> (22.9289, 40)
  line L730 (42.9289, 40) -> (40, 37.0711)
  line L731 (40, 37.0711) -> (37.0711, 40)
  line L732 (37.0711, 40) -> (40, 42.9289)
  line L733 (40, 42.9289) -> (42.9289, 40)
  line L734 (42.9289, 30) -> (40, 27.0711)
  line L735 (40, 27.0711) -> (37.0711, 30)
  line L736 (37.0711, 30) -> (40, 32.9289)
  line L737 (40, 32.9289) -> (42.9289, 30)
  line L738 (12.9289, 50) -> (10, 47.0711)
  line L739 (10, 47.0711) -> (7.0711, 50)
  line L740 (7.0711, 50) -> (10, 52.9289)
  line L741 (10, 52.9289) -> (12.9289, 50)
  line L742 (42.9289, 50) -> (40, 47.0711)
  line L743 (40, 47.0711) -> (37.0711, 50)
  line L744 (37.0711, 50) -> (40, 52.9289)
  line L745 (40, 52.9289) -> (42.9289, 50)
  line L746 (32.9289, 50) -> (30, 47.0711)
  line L747 (30, 47.0711) -> (27.0711, 50)
  line L748 (27.0711, 50) -> (30, 52.9289)
  line L749 (30, 52.9289) -> (32.9289, 50)
  line L750 (22.9289, 50) -> (20, 47.0711)
  line L751 (20, 47.0711) -> (17.0711, 50)
  line L752 (17.0711, 50) -> (20, 52.9289)
  line L753 (20, 52.9289) -> (22.9289, 50)
  line L754 (52.9289, 50) -> (50, 47.0711)
  line L755 (50, 47.0711) -> (47.0711, 50)
  line L756 (47.0711, 50) -> (50, 52.9289)
  line L757 (50, 52.9289) -> (52.9289, 50)
  line L758 (52.9289, 40) -> (50, 37.0711)
  line L759 (50, 37.0711) -> (47.0711, 40)
  line L760 (47.0711, 40) -> (50, 42.9289)
  line L761 (50, 42.9289) -> (52.9289, 40)
  line L762 (12.9289, 60) -> (10, 57.0711)
  line L763 (10, 57.0711) -> (7.0711, 60)
  line L764 (7.0711, 60) -> (10, 62.9289)
  line L765 (10, 62.9289) -> (12.9289, 60)
  line L766 (52.9289, 30) -> (50, 27.0711)
  line L767 (50, 27.0711) -> (47.0711, 30)
  line L768 (47.0711, 30) -> (50, 32.9289)
  line L769 (50, 32.9289) -> (52.9289, 30)
  line L770 (22.9289, 60) -> (20, 57.0711)
  line L771 (20, 57.0711) -> (17.0711, 60)
  line L772 (17.0711, 60) -> (20, 62.9289)
  line L773 (20, 62.9289) -> (22.9289, 60)
  line L774 (42.9289, 60) -> (40, 57.0711)
  line L775 (40, 57.0711) -> (37.0711, 60)
  line L776 (37.0711, 60) -> (40, 62.9289)
  line L777 (40, 62.9289) -> (42.9289, 60)
  line L778 (52.9289, 60) -> (50, 57.0711)
  line L779 (50, 57.0711) -> (47.0711, 60)
  line L780 (47.0711, 60) -> (50, 62.9289)
  line L781 (50, 62.9289) -> (52.9289, 60)
  line L782 (32.9289, 60) -> (30, 57.0711)
  line L783 (30, 57.0711) -> (27.0711, 60)
  line L784 (27.0711, 60) -> (30, 62.9289)
  line L785 (30, 62.9289) -> (32.9289, 60)
  line L786 (62.9289, 60) -> (60, 57.0711)
  line L787 (60, 57.0711) -> (57.0711, 60)
  line L788 (57.0711, 60) -> (60, 62.9289)
  line L789 (60, 62.9289) -> (62.9289, 60)
  line L790 (62.9289, 40) -> (60, 37.0711)
  line L791 (60, 37.0711) -> (57.0711, 40)
  line L792 (57.0711, 40) -> (60, 42.9289)
  line L793 (60, 42.9289) -> (62.9289, 40)
  line L794 (62.9289, 50) -> (60, 47.0711)
  line L795 (60, 47.0711) -> (57.0711, 50)
  line L796 (57.0711, 50) -> (60, 52.9289)
  line L797 (60, 52.9289) -> (62.9289, 50)
  line L798 (21, 3.3431) -> (21, 6.6569)
  line L799 (21, 6.6569) -> (23.3431, 9)
  line L800 (23.3431, 9) -> (26.6569, 9)
  line L801 (26.6569, 9) -> (29, 6.6569)
  line L802 (29, 6.6569) -> (29, 3.3431)
  line L803 (29, 3.3431) -> (26.6569, 1)
  line L804 (26.6569, 1) -> (23.3431, 1)
  line L805 (23.3431, 1) -> (21, 3.3431)
  line L806 (41, -6.6569) -> (41, -3.3431)
  line L807 (41, -3.3431) -> (43.3431, -1)
  line L808 (43.3431, -1) -> (46.6569, -1)
  line L809 (46.6569, -1) -> (49, -3.3431)
  line L810 (49, -3.3431) -> (49, -6.6569)
  line L811 (49, -6.6569) -> (46.6569, -9)
  line L812 (46.6569, -9) -> (43.3431, -9)
  line L813 (43.3431, -9) -> (41, -6.6569)
  line L814 (-59, 13.3431) -> (-59, 16.6569)
  line L815 (-59, 16.6569) -> (-56.6569, 19)
  line L816 (-56.6569, 19) -> (-53.3431, 19)
  line L817 (-53.3431, 19) -> (-51, 16.6569)
  line L818 (-51, 16.6569) -> (-51, 13.3431)
  line L819 (-51, 13.3431) -> (-53.3431, 11)
  line L820 (-53.3431, 11) -> (-56.6569, 11)
  line L821 (-56.6569, 11) -> (-59, 13.3431)
  line L822 (11, 3.3431) -> (11, 6.6569)
  line L823 (11, 6.6569) -> (13.3431, 9)
  line L824 (13.3431, 9) -> (16.6569, 9)
  line L825 (16.6569, 9) -> (19, 6.6569)
  line L826 (19, 6.6569) -> (19, 3.3431)
  line L827 (19, 3.3431) -> (16.6569, 1)
  line L828 (16.6569, 1) -> (13.3431, 1)
  line L829 (13.3431, 1) -> (11, 3.3431)
  line L830 (-69, 13.3431) -> (-69, 16.6569)
  line L831 (-69, 16.6569) -> (-66.6569, 19)
  line L832 (-66.6569, 19) -> (-63.3431, 19)
  line L833 (-63.3431, 19) -> (-61, 16.6569)
  line L834 (-61, 16.6569) -> (-61, 13.3431)
  line L835 (-61, 13.3431) -> (-63.3431, 11)
  line L836 (-63.3431, 11) -> (-66.6569, 11)
  line L837 (-66.6569, 11) -> (-69, 13.3431)
  line L838 (-49, 13.3431) -> (-49, 16.6569)
  line L839 (-49, 16.6569) -> (-46.6569, 19)
  line L840 (-46.6569, 19) -> (-43.3431, 19)
  line L841 (-43.3431, 19) -> (-41, 16.6569)
  line L842 (-41, 16.6569) -> (-41, 13.3431)
  line L843 (-41, 13.3431) -> (-43.3431, 11)
  line L844 (-43.3431, 11) -> (-46.6569, 11)
  line L845 (-46.6569, 11) -> (-49, 13.3431)
  line L846 (-49, 3.3431) -> (-49, 6.6569)
  line L847 (-49, 6.6569) -> (-46.6569, 9)
  line L848 (-46.6569, 9) -> (-43.3431, 9)
  line L849 (-43.3431, 9) -> (-41, 6.6569)
  line L850 (-41, 6.6569) -> (-41, 3.3431)
  line L851 (-41, 3.3431) -> (-43.3431, 1)
  line L852 (-43.3431, 1) -> (-46.6569, 1)
  line L853 (-46.6569, 1) -> (-49, 3.3431)
  line L854 (11, -6.6569) -> (11, -3.3431)
  line L855 (11, -3.3431) -> (13.3431, -1)
  line L856 (13.3431, -1) -> (16.6569, -1)
  line L857 (16.6569, -1) -> (19, -3.3431)
  line L858 (19, -3.3431) -> (19, -6.6569)
  line L859 (19, -6.6569) -> (16.6569, -9)
  line L860 (16.6569, -9) -> (13.3431, -9)
  line L861 (13.3431, -9) -> (11, -6.6569)
  line L862 (61, 3.3431) -> (61, 6.6569)
  line L863 (61, 6.6569) -> (63.3431, 9)
  line L864 (63.3431, 9) -> (66.6569, 9)
  line L865 (66.6569, 9) -> (69, 6.6569)
  line L866 (69, 6.6569) -> (69, 3.3431)
  line L867 (69, 3.3431) -> (66.6569, 1)
  line L868 (66.6569, 1) -> (63.3431, 1)
  line L869 (63.3431, 1) -> (61, 3.3431)
  line L870 (51, 3.3431) -> (51, 6.6569)
  line L871 (51, 6.6569) -> (53.3431, 9)
  line L872 (53.3431, 9) -> (56.6569, 9)
  line L873 (56.6569, 9) -> (59, 6.6569)
  line L874 (59, 6.6569) -> (59, 3.3431)
  line L875 (59, 3.3431) -> (56.6569, 1)
  line L876 (56.6569, 1) -> (53.3431, 1)
  line L877 (53.3431, 1) -> (51, 3.3431)
  line L878 (31, -6.6569) -> (31, -3.3431)
  line L879 (31, -3.3431) -> (33.3431, -1)
  line L880 (33.3431, -1) -> (36.6569, -1)
  line L881 (36.6569, -1) -> (39, -3.3431)
  line L882 (39, -3.3431) -> (39, -6.6569)
  line L883 (39, -6.6569) -> (36.6569, -9)
  line L884 (36.6569, -9) -> (33.3431, -9)
  line L885 (33.3431, -9) -> (31, -6.6569)
  line L886 (21, -6.6569) -> (21, -3.3431)
  line L887 (21, -3.3431) -> (23.3431, -1)
  line L888 (23.3431, -1) -> (26.6569, -1)
  line L889 (26.6569, -1) -> (29, -3.3431)
  line L890 (29, -3.3431) -> (29, -6.6569)
  line L891 (29, -6.6569) -> (26.6569, -9)
  line L892 (26.6569, -9) -> (23.3431, -9)
  line L893 (23.3431, -9) -> (21, -6.6569)
  line L894 (41, 3.3431) -> (41, 6.6569)
  line L895 (41, 6.6569) -> (43.3431, 9)
  line L896 (43.3431, 9) -> (46.6569, 9)
  line L897 (46.6569, 9) -> (49, 6.6569)
  line L898 (49, 6.6569) -> (49, 3.3431)
  line L899 (49, 3.3431) -> (46.6569, 1)
  line L900 (46.6569, 1) -> (43.3431, 1)
  line L901 (43.3431, 1) -> (41, 3.3431)
  line L902 (-29, 13.3431) -> (-29, 16.6569)
  line L903 (-29, 16.6569) -> (-26.6569, 19)
  line L904 (-26.6569, 19) -> (-23.3431, 19)
  line L905 (-23.3431, 19) -> (-21, 16.6569)
  line L906 (-21, 16.6569) -> (-21, 13.3431)
  line L907 (-21, 13.3431) -> (-23.3431, 11)
  line L908 (-23.3431, 11) -> (-26.6569, 11)
  line L909 (-26.6569, 11) -> (-29, 13.3431)
  line L910 (1, 3.3431) -> (1, 6.6569)
  line L911 (1, 6.6569) -> (3.3431, 9)
  line L912 (3.3431, 9) -> (6.6569, 9)
  line L913 (6.6569, 9) -> (9, 6.6569)
  line L914 (9, 6.6569) -> (9, 3.3431)
  line L915 (9, 3.3431) -> (6.6569, 1)
  line L916 (6.6569, 1) -> (3.3431, 1)
  line L917 (3.3431, 1) -> (1, 3.3431)
  line L918 (-9, 3.3431) -> (-9, 6.6569)
  line L919 (-9, 6.6569) -> (-6.6569, 9)
  line L920 (-6.6569, 9) -> (-3.3431, 9)
  line L921 (-3.3431, 9) -> (-1, 6.6569)
  line L922 (-1, 6.6569) -> (-1, 3.3431)
  line L923 (-1, 3.3431) -> (-3.3431, 1)
  line L924 (-3.3431, 1) -> (-6.6569, 1)
  line L925 (-6.6569, 1) -> (-9, 3.3431)
  line L926 (-19, 13.3431) -> (-19, 16.6569)
  line L927 (-19, 16.6569) -> (-16.6569, 19)
  line L928 (-16.6569, 19) -> (-13.3431, 19)
  line L929 (-13.3431, 19) -> (-11, 16.6569)
  line L930 (-11, 16.6569) -> (-11, 13.3431)
  line L931 (-11, 13.3431) -> (-13.3431, 11)
  line L932 (-13.3431, 11) -> (-16.6569, 11)
  line L933 (-16.6569, 11) -> (-19, 13.3431)
  line L934 (-29, 3.3431) -> (-29, 6.6569)
  line L935 (-29, 6.6569) -> (-26.6569, 9)
  line L936 (-26.6569, 9) -> (-23.3431, 9)
  line L937 (-23.3431, 9) -> (-21, 6.6569)
  line L938 (-21, 6.6569) -> (-21, 3.3431)
  line L939 (-21, 3.3431) -> (-23.3431, 1)
  line L940 (-23.3431, 1) -> (-26.6569, 1)
  line L941 (-26.6569, 1) -> (-29, 3.3431)
  line L942 (-69, 3.3431) -> (-69, 6.6569)
  line L943 (-69, 6.6569) -> (-66.6569, 9)
  line L944 (-66.6569, 9) -> (-63.3431, 9)
  line L945 (-63.3431, 9) -> (-61, 6.6569)
  line L946 (-61, 6.6569) -> (-61, 3.3431)
  line L947 (-61, 3.3431) -> (-63.3431, 1)
  line L948 (-63.3431, 1) -> (-66.6569, 1)
  line L949 (-66.6569, 1) -> (-69, 3.3431)
  line L950 (31, 3.3431) -> (31, 6.6569)
  line L951 (31, 6.6569) -> (33.3431, 9)
  line L952 (33.3431, 9) -> (36.6569, 9)
  line L953 (36.6569, 9) -> (39, 6.6569)
  line L954 (39, 6.6569) -> (39, 3.3431)
  line L955 (39, 3.3431) -> (36.6569, 1)
  line L956 (36.6569, 1) -> (33.3431, 1)
  line L957 (33.3431, 1) -> (31, 3.3431)
  line L958 (-59, 3.3431) -> (-59, 6.6569)
  line L959 (-59, 6.6569) -> (-56.6569, 9)
  line L960 (-56.6569, 9) -> (-53.3431, 9)
  line L961 (-53.3431, 9) -> (-51, 6.6569)
  line L962 (-51, 6.6569) -> (-51, 3.3431)
  line L963 (-51, 3.3431) -> (-53.3431, 1)
  line L964 (-53.3431, 1) -> (-56.6569, 1)
  line L965 (-56.6569, 1) -> (-59, 3.3431)
  line L966 (61, -6.6569) -> (61, -3.3431)
  line L967 (61, -3.3431) -> (63.3431, -1)
  line L968 (63.3431, -1) -> (66.6569, -1)
  line L969 (66.6569, -1) -> (69, -3.3431)
  line L970 (69, -3.3431) -> (69, -6.6569)
  line L971 (69, -6.6569) -> (66.6569, -9)
  line L972 (66.6569, -9) -> (63.3431, -9)
  line L973 (63.3431, -9) -> (61, -6.6569)
  line L974 (1, -6.6569) -> (1, -3.3431)
  line L975 (1, -3.3431) -> (3.3431, -1)
  line L976 (3.3431, -1) -> (6.6569, -1)
  line L977 (6.6569, -1) -> (9, -3.3431)
  line L978 (9, -3.3431) -> (9, -6.6569)
  line L979 (9, -6.6569) -> (6.6569, -9)
  line L980 (6.6569, -9) -> (3.3431, -9)
  line L981 (3.3431, -9) -> (1, -6.6569)
  line L982 (51, -6.6569) -> (51, -3.3431)
  line L983 (51, -3.3431) -> (53.3431, -1)
  line L984 (53.3431, -1) -> (56.6569, -1)
  line L985 (56.6569, -1) -> (59, -3.3431)
  line L986 (59, -3.3431) -> (59, -6.6569)
  line L987 (59, -6.6569) -> (56.6569, -9)
  line L988 (56.6569, -9) -> (53.3431, -9)
  line L989 (53.3431, -9) -> (51, -6.6569)
  line L990 (-39, 3.3431) -> (-39, 6.6569)
  line L991 (-39, 6.6569) -> (-36.6569, 9)
  line L992 (-36.6569, 9) -> (-33.3431, 9)
  line L993 (-33.3431, 9) -> (-31, 6.6569)
  line L994 (-31, 6.6569) -> (-31, 3.3431)
  line L995 (-31, 3.3431) -> (-33.3431, 1)
  line L996 (-33.3431, 1) -> (-36.6569, 1)
  line L997 (-36.6569, 1) -> (-39, 3.3431)
  line L998 (-19, 3.3431) -> (-19, 6.6569)
  line L999 (-19, 6.6569) -> (-16.6569, 9)
  line L1000 (-16.6569, 9) -> (-13.3431, 9)
  line L1001 (-13.3431, 9) -> (-11, 6.6569)
  line L1002 (-11, 6.6569) -> (-11, 3.3431)
  line L1003 (-11, 3.3431) -> (-13.3431, 1)
  line L1004 (-13.3431, 1) -> (-16.6569, 1)
  line L1005 (-16.6569, 1) -> (-19, 3.3431)
  line L1006 (32.9289, -60) -> (30, -62.9289)
  line L1007 (30, -62.9289) -> (27.0711, -60)
  line L1008 (27.0711, -60) -> (30, -57.0711)
  line L1009 (30, -57.0711) -> (32.9289, -60)
  line L1010 (42.9289, -60) -> (40, -62.9289)
  line L1011 (40, -62.9289) -> (37.0711, -60)
  line L1012 (37.0711, -60) -> (40, -57.0711)
  line L1013 (40, -57.0711) -> (42.9289, -60)
  line L1014 (52.9289, -60) -> (50, -62.9289)
  line L1015 (50, -62.9289) -> (47.0711, -60)
  line L1016 (47.0711, -60) -> (50, -57.0711)
  line L1017 (50, -57.0711) -> (52.9289, -60)
  line L1018 (62.9289, -60) -> (60, -62.9289)
  line L1019 (60, -62.9289) -> (57.0711, -60)
  line L1020 (57.0711, -60) -> (60, -57.0711)
  line L1021 (60, -57.0711) -> (62.9289, -60)
  line L1022 (62.9289, -50) -> (60, -52.9289)
  line L1023 (60, -52.9289) -> (57.0711, -50)
  line L1024 (57.0711, -50) -> (60, -47.0711)
  line L1025 (60, -47.0711) -> (62.9289, -50)
  line L1026 (62.9289, -40) -> (60, -42.9289)
  line L1027 (60, -42.9289) -> (57.0711, -40)
  line L1028 (57.0711, -40) -> (60, -37.0711)
  line L1029 (60, -37.0711) -> (62.9289, -40)
  line L1030 (62.9289, -30) -> (60, -32.9289)
  line L1031 (60, -32.9289) -> (57.0711, -30)
  line L1032 (57.0711, -30) -> (60, -27.0711)
  line L1033 (60, -27.0711) -> (62.9289, -30)
  line L1034 (62.9289, -20) -> (60, -22.9289)
  line L1035 (60, -22.9289) -> (57.0711, -20)
  line L1036 (57.0711, -20) -> (60, -17.0711)
  line L1037 (60, -17.0711) -> (62.9289, -20)
  line L1038 (62.9289, -10) -> (60, -12.9289)
  line L1039 (60, -12.9289) -> (57.0711, -10)
  line L1040 (57.0711, -10) -> (60, -7.0711)
  line L1041 (60, -7.0711) -> (62.9289, -10)
  line L1042 (62.9289, 10) -> (60, 7.0711)
  line L1043 (60, 7.0711) -> (57.0711, 10)
  line L1044 (57.0711, 10) -> (60, 12.9289)
  line L1045 (60, 12.9289) -> (62.9289, 10)
  line L1046 (62.9289, 0) -> (60, -2.9289)
  line L1047 (60, -2.9289) -> (57.0711, 0)
  line L1048 (57.0711, 0) -> (60, 2.9289)
  line L1049 (60, 2.9289) -> (62.9289, 0)
  line L1050 (62.9289, 20) -> (60, 17.0711)
  line L1051 (60, 17.0711) -> (57.0711, 20)
  line L1052 (57.0711, 20) -> (60, 22.9289)
  line L1053 (60, 22.9289) -> (62.9289, 20)
  line L1054 (-37.0711, 60) -> (-40, 57.0711)
  line L1055 (-40, 57.0711) -> (-42.9289, 60)
  line L1056 (-42.9289, 60) -> (-40, 62.9289)
  line L1057 (-40, 62.9289) -> (-37.0711, 60)
  line L1058 (2.9289, 60) -> (0, 57.0711)
  line L1059 (0, 57.0711) -> (-2.9289, 60)
  line L1060 (-2.9289, 60) -> (0, 62.9289)
  line L1061 (0, 62.9289) -> (2.9289, 60)
  line L1062 (-27.0711, 60) -> (-30, 57.0711)
  line L1063 (-30, 57.0711) -> (-32.9289, 60)
  line L1064 (-32.9289, 60) -> (-30, 62.9289)
  line L1065 (-30, 62.9289) -> (-27.0711, 60)
  line L1066 (-17.0711, 60) -> (-20, 57.0711)
  line L1067 (-20, 57.0711) -> (-22.9289, 60)
  line L1068 (-22.9289, 60) -> (-20, 62.9289)
  line L1069 (-20, 62.9289) -> (-17.0711, 60)
  line L1070 (-7.0711, 60) -> (-10, 57.0711)
  line L1071 (-10, 57.0711) -> (-12.9289, 60)
  line L1072 (-12.9289, 60) -> (-10, 62.9289)
  line L1073 (-10, 62.9289) -> (-7.0711, 60)
  line L1074 (12.9289, -60) -> (10, -62.9289)
  line L1075 (10, -62.9289) -> (7.0711, -60)
  line L1076 (7.0711, -60) -> (10, -57.0711)
  line L1077 (10, -57.0711) -> (12.9289, -60)
  line L1078 (22.9289, -60) -> (20, -62.9289)
  line L1079 (20, -62.9289) -> (17.0711, -60)
  line L1080 (17.0711, -60) -> (20, -57.0711)
  line L1081 (20, -57.0711) -> (22.9289, -60)
  line L1082 (2.9289, -60) -> (0, -62.9289)
  line L1083 (0, -62.9289) -> (-2.9289, -60)
  line L1084 (-2.9289, -60) -> (0, -57.0711)
  line L1085 (0, -57.0711) -> (2.9289, -60)
  line L1086 (-17.0711, -50) -> (-20, -52.9289)
  line L1087 (-20, -52.9289) -> (-22.9289, -50)
  line L1088 (-22.9289, -50) -> (-20, -47.0711)
  line L1089 (-20, -47.0711) -> (-17.0711, -50)
  line L1090 (-7.0711, -60) -> (-10, -62.9289)
  line L1091 (-10, -62.9289) -> (-12.9289, -60)
  line L1092 (-12.9289, -60) -> (-10, -57.0711)
  line L1093 (-10, -57.0711) -> (-7.0711, -60)
  line L1094 (-37.0711, -60) -> (-40, -62.9289)
  line L1095 (-40, -62.9289) -> (-42.9289, -60)
  line L1096 (-42.9289, -60) -> (-40, -57.0711)
  line L1097 (-40, -57.0711) -> (-37.0711, -60)
  line L1098 (-27.0711, -50) -> (-30, -52.9289)
  line L1099 (-30, -52.9289) -> (-32.9289, -50)
  line L1100 (-32.9289, -50) -> (-30, -47.0711)
  line L1101 (-30, -47.0711) -> (-27.0711, -50)
  line L1102 (-27.0711, -60) -> (-30, -62.9289)
  line L1103 (-30, -62.9289) -> (-32.9289, -60)
  line L1104 (-32.9289, -60) -> (-30, -57.0711)
  line L1105 (-30, -57.0711) -> (-27.0711, -60)
  line L1106 (-17.0711, -60) -> (-20, -62.9289)
  line L1107 (-20, -62.9289) -> (-22.9289, -60)
  line L1108 (-22.9289, -60) -> (-20, -57.0711)
  line L1109 (-20, -57.0711) -> (-17.0711, -60)
  line L1110 (-7.0711, 10) -> (-10, 7.0711)
  line L1111 (-10, 7.0711) -> (-12.9289, 10)
  line L1112 (-12.9289, 10) -> (-10, 12.9289)
  line L1113 (-10, 12.9289) -> (-7.0711, 10)
  line L1114 (-7.0711, 0) -> (-10, -2.9289)
  line L1115 (-10, -2.9289) -> (-12.9289, 0)
  line L1116 (-12.9289, 0) -> (-10, 2.9289)
  line L1117 (-10, 2.9289) -> (-7.0711, 0)
  line L1118 (12.9289, 10) -> (10, 7.0711)